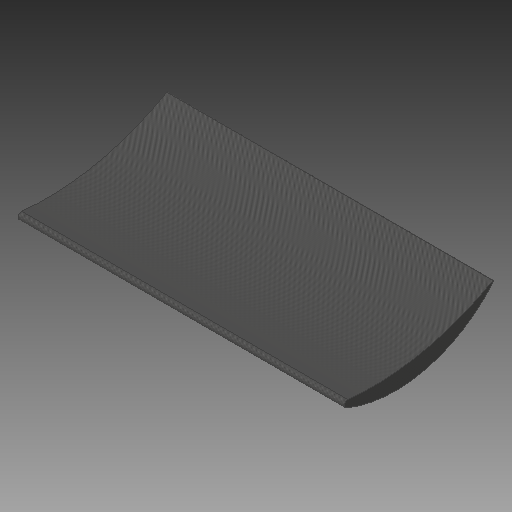
# Autodesk Inventor part: cover_re
Saved by Autodesk Inventor 2018.1 (Build 221171000, 171)
## iProperties
Created: 2017-10-27
Part Number: cover_re
Material: CFRP
Document SubType Name: Modeling
Designer: kuwano
Density: 1.43 g/cm^3
Appearance: カーボンファイバー
Author: kuwano
Autodesk Inventor part; units mm, degrees
ref_plane "YZ Plane" through (0, 0, 0) normal (1, 0, 0) x (0, 1, 0)
ref_plane "XZ Plane" through (0, 0, 0) normal (0, 1, 0) x (-1, 0, 0)
ref_plane "XY Plane" through (0, 0, 0) normal (0, 0, 1) x (1, 0, 0)
sketch "スケッチ1" plane through (0, 0, 0) normal (1, 0, 0) x (0, 1, 0)
  line L0 (0, 250) -> (88.1635, -250)
  line L1 (0, 353.3532) -> (0, -370.1192) projected
  arc A0 (0, 250) -> (88.1635, -250) centre (710.7652, 117.5543) ccw
  arc A1 (0, 250) -> (88.1635, -250) centre (325.1936, 49.5676) ccw
  point P0 (0, 0)
  dimension "d0" = 10
  dimension "d1" = 500
  dimension "d2" = 723
  dimension "d3" = 382
  dimension "d4" = 250
  constraints: 4 point on circle, 2 centre point, 2 end point, 1 point on line
  measures "d0" angle of L1 L0
  measures "d1" vertical distance of L0.end L0.start
  measures "d2" radius of A0
  measures "d3" radius of A1
  measures "d4" distance of point (0, 0) L0.start
extrude "押し出し1" add sketch "スケッチ1" along normal mid plane 970 contours A0 L1 A1 | A1 L1 A0
fillet "フィレット1" radius 10 1 edges at (0, 0, 250)
fillet "フィレット2" radius 2 1 edges at (0, 88.1635, -250)
